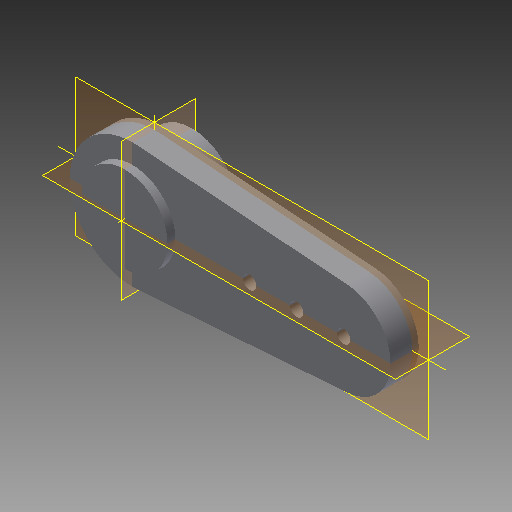
# Autodesk Inventor part: ASV-15MGSingleHorn01
Saved by Autodesk Inventor 2017.3 (Build 213256000, 256)
## iProperties
Created: 2015-02-16
Part Number: ASV-15MGSingleHorn01
Material: 一般
Document SubType Name: Modeling
Designer: Yamaura
Density: 1 g/cm^3
Appearance: 既定
Author: Yamaura
Autodesk Inventor part; units mm, degrees
sketch "スケッチ1" plane through (0, 0, 0) normal (0, 0, 1) x (1, 0, 0)
  circle A0 centre (0, 0) radius 2.875
  dimension "d0" = 5.75
  constraints: 1 centre point, 1 coincident
  measures "d0" diameter of A0
extrude "押し出し1" add sketch "スケッチ1" against normal blind 2.4
sketch "スケッチ2" plane through (0, 0, 0) normal (0, 0, 1) x (1, 0, 0)
  circle A0 centre (0, 0) radius 2.75
  dimension "d3" = 5.5
  constraints: 1 centre point, 1 coincident
  measures "d3" diameter of A0
extrude "押し出し2" add sketch "スケッチ2" along normal blind 1.9
sketch "スケッチ3" plane through (0, 0, 0) normal (0, 0, 1) x (1, 0, 0)
  circle A0 centre (0, 0) radius 4
  circle A1 centre (13.5, 0) radius 3
  line L0 (-5.7629, 0) -> (13.5774, 0) projected
  line L1 (0.2963, 3.989) -> (13.7222, 2.9918)
  line L2 (13.7222, -2.9918) -> (0.2963, -3.989)
  dimension "d6" = 8
  dimension "d7" = 6
  dimension "d8" = 13.5
  constraints: 4 end point, 4 point on circle, 4 tangent, 2 centre point, 1 coincident, 1 point on line
  measures "d6" diameter of A0
  measures "d7" diameter of A1
  measures "d8" distance of point (0, 0) A1.centre
extrude "押し出し3" add sketch "スケッチ3" along normal blind 1.4 and the other way blind 0.4
sketch "スケッチ4" plane through (0, 0, 0) normal (0, 0, 1) x (1, 0, 0)
  circle A0 centre (13.5, 0) radius 0.43
  point P0 (0, 0)
  dimension "d13" = 0.86
  dimension "d15" = 13.5
  constraints: 1 centre point
  measures "d13" diameter of A0
  measures "d15" distance of A0.centre point (0, 0)
extrude "押し出し4" cut sketch "スケッチ4" along normal through all both and the other way through all
sketch "スケッチ5" plane through (0, 0, 0) normal (0, 0, 1) x (1, 0, 0)
  circle A0 centre (0, 0) radius 1.9
  dimension "d22" = 3.8
  constraints: 1 centre point, 1 coincident
  measures "d22" diameter of A0
extrude "押し出し5" cut sketch "スケッチ5" against normal through all
pattern_linear "矩形状パターン1" count 3 spacing 3 along (-1, 0, 0) of "押し出し4"
